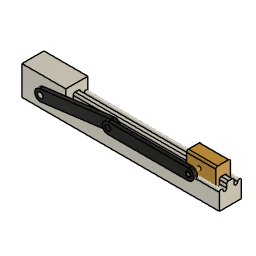
Simple Joint Mechanism_ (Autodesk Fusion 360 design; units mm, degrees)
Autodesk Fusion 360 part; units mm, degrees
sketch "Sketch1" plane through (0, 0, 0) normal (0, 1, 0) x (1, 0, 0) in component "block"
  line L0 (0, 0) -> (120, 0)
  line L1 (120, 0) -> (120, -80)
  line L2 (120, -80) -> (0, -80)
  line L3 (0, -80) -> (0, 0)
  line L4 (120, 0) -> (540, 0)
  line L5 (540, 0) -> (540, -50)
  line L6 (540, -50) -> (120, -50)
  line L7 (120, -50) -> (120, 0)
  dimension "d1" = 120
  dimension "d2" = 80
  dimension "d3" = 420
  dimension "d4" = 50
  constraint horizontal L0
  constraint vertical L1
  constraint horizontal L2
  constraint vertical L3
  constraint coincident L0.start L3.end
  constraint horizontal L4
  constraint vertical L5
  constraint horizontal L6
  constraint vertical L7
  measures "d1" distance of L0.start L0.end
  measures "d2" distance of L0.start L2.end
  measures "d3" distance of L0.end L4.end
  measures "d4" distance of L0.end L6.end
extrude "Extrude1" add sketch "Sketch1" along normal mid plane 60 makes body 1 in component "block"
sketch "Sketch2" plane through (120, 0, 0) normal (1, 0, 0) x (0, 1, 0) in component "block"
  line L0 (-30, 50) -> (30, 50)
  line L1 (30, 50) -> (30, 80)
  line L2 (30, 80) -> (-30, 80)
  line L3 (-30, 80) -> (-30, 50)
  line L4 (-10, 50) -> (10, 50)
  line L5 (10, 50) -> (10, 60)
  line L6 (10, 60) -> (-10, 60)
  line L7 (-10, 60) -> (-10, 50)
  line L8 (-10, 50) -> (-20, 50)
  line L9 (-20, 50) -> (-20, 40)
  line L10 (-20, 40) -> (-10, 40)
  line L11 (-10, 40) -> (-10, 50)
  line L12 (10, 50) -> (20, 50)
  line L13 (20, 50) -> (20, 40)
  line L14 (20, 40) -> (10, 40)
  line L15 (10, 40) -> (10, 50)
  dimension "d7" = 20
  dimension "d8" = 10
  dimension "d9" = 10
  dimension "d10" = 10
  dimension "d11" = 10
  dimension "d12" = 10
  constraint horizontal L4
  constraint vertical L5
  constraint horizontal L6
  constraint vertical L7
  constraint coincident L0 L4.start
  constraint horizontal L8
  constraint vertical L9
  constraint horizontal L10
  constraint vertical L11
  constraint horizontal L12
  constraint vertical L13
  constraint horizontal L14
  constraint vertical L15
  measures "d7" distance of L4.start L4.end
  measures "d8" distance of L4.start L6.end
  measures "d9" distance of L4.start L8.end
  measures "d10" distance of L4.start L10.end
  measures "d11" distance of L4.end L12.end
  measures "d12" distance of L4.end L14.end
extrude "Extrude2" add sketch "Sketch2" along normal blind 420 contours L0 L4 L5 L6 L7 bodies 1 in component "block"
extrude "Extrude3" cut sketch "Sketch2" along normal blind 420 contours L0 L8 L9 L10 L11 | L0 L12 L13 L14 L15 bodies 1 in component "block"
fillet "Fillet1" radius 5 9 edges at (330, -30, 50) (330, -20, 50) (330, -20, 40) (330, -10, 60) (330, 10, 60) (330, 10, 40) (330, 20, 40) (330, 20, 50) (330, 30, 50) on bodies 1 in component "block"
sketch "Sketch3" plane through (0, 30, 0) normal (0, 1, 0) x (-1, 0, 0) in component "block"
  line L0 (-120, 45) -> (-540, 45)
  line L1 (-540, 45) -> (-540, 0)
  line L2 (-540, 0) -> (0, 0)
  line L3 (0, 0) -> (0, 80)
  line L4 (0, 80) -> (-120, 80)
  line L5 (-120, 80) -> (-120, 45)
  circle A0 centre (-60, 40) radius 7.5
  dimension "d19" = 15
  dimension "d20" = 60
  dimension "d21" = 40
  measures "d19" diameter of A0
  measures "d20" horizontal distance of L2.end A0.centre
  measures "d21" vertical distance of L2.end A0.centre
extrude "Extrude4" add sketch "Sketch3" against normal blind 70 contours A0 bodies 1 in component "block"
sketch "Sketch1 (2)" plane through (0, -30, 0) normal (0, -1, 0) x (1, 0, 0) in component "arm1"
  circle A0 centre (60, 40) radius 7.5
  line L0 (540, 45) -> (120, 45)
  line L1 (120, 45) -> (120, 80)
  line L2 (120, 80) -> (0, 80)
  line L3 (0, 80) -> (0, 0)
  line L4 (0, 0) -> (540, 0)
  line L5 (540, 0) -> (540, 45)
  circle A1 centre (60, 40) radius 7.5
  line L6 (38.7868, 40) -> (60, 18.7868)
  line L7 (60, 18.7868) -> (220, 178.7868)
  line L8 (220, 178.7868) -> (198.7868, 200)
  line L9 (198.7868, 200) -> (38.7868, 40)
  circle A2 centre (198.7868, 178.7868) radius 7.5
  dimension "d24" = 15
  dimension "d25" = 15
  dimension "d26" = 30
  dimension "d27" = 160
  dimension "d28" = 15
  dimension "d29" = 15
  dimension "d30" = 15
  constraint perpendicular L6 L7
  constraint parallel L6 L8
  constraint parallel L7 L9
  measures "d24" distance of A0.centre L6
  measures "d25" distance of A0.centre L7
  measures "d26" distance of L6.start L6.end
  measures "d27" vertical distance of L6.start L8.end
  measures "d28" diameter of A2
  measures "d29" distance of L7 A2.centre
  measures "d30" distance of L8 A2.centre
extrude "Extrude1'" add sketch "Sketch1 (2)" along normal blind 10 separate body contours L1 L2 L6 L7 L9 | L1 L2 L7 L8 L9 makes body 2 in component "arm1"
fillet "Fillet1'" radius 15 4 edges at (220, -35, 178.7868) (198.7868, -35, 200) (38.7868, -35, 40) (60, -35, 18.7868) on bodies 2 in component "arm1"
extrude "Extrude2'" add sketch "Sketch1 (2)" along normal blind 20 contours A2 bodies 2 in component "arm1"
sketch "Sketch1 (3)" plane through (540, 0, 0) normal (1, 0, 0) x (0, 1, 0) in component "slide"
  arc A0 (30, 45) -> (20, 45) centre (25, 45) ccw
  arc A1 (10, 45) -> (20, 45) centre (15, 45) ccw
  line L0 (10, 45) -> (10, 55)
  arc A2 (10, 55) -> (5, 60) centre (5, 55) ccw
  line L1 (5, 60) -> (-5, 60)
  arc A3 (-5, 60) -> (-10, 55) centre (-5, 55) ccw
  line L2 (-10, 55) -> (-10, 40)
  line L3 (-10, 40) -> (-15, 40)
  arc A4 (-20, 45) -> (-15, 40) centre (-15, 45) ccw
  arc A5 (-20, 45) -> (-30, 45) centre (-25, 45) ccw
  line L4 (-30, 45) -> (-30, 0)
  line L5 (-30, 0) -> (30, 0)
  line L6 (30, 0) -> (30, 45)
  line L7 (-20, 39.856) -> (20, 39.856)
  line L8 (20, 39.856) -> (20, 89.856)
  line L9 (20, 89.856) -> (-20, 89.856)
  line L10 (-20, 89.856) -> (-20, 39.856)
  dimension "d48" = 40
  dimension "d49" = 50
  constraint horizontal L7
  constraint vertical L8
  constraint horizontal L9
  constraint vertical L10
  measures "d48" distance of L7.start L7.end
  measures "d49" distance of L7.start L9.end
extrude "Extrude1''" add sketch "Sketch1 (3)" against normal blind 80 separate body contours A1 L0 A2 L1 A3 L2 L3 A4 L8 L9 L10 makes body 3 in component "slide"
fillet "Fillet1''" radius 5 2 edges at (500, 20, 89.856) (500, -20, 89.856) on bodies 3 in component "slide"
fillet "Fillet2" radius 5 1 edges at (330, -10, 40) on bodies 1 in component "block"
sketch "Sketch2 (2)" plane through (0, -20, 0) normal (0, -1, 0) x (1, 0, 0) in component "slide"
  line L0 (540, 84.856) -> (460, 84.856)
  line L1 (460, 84.856) -> (460, 45)
  line L2 (460, 45) -> (540, 45)
  line L3 (540, 45) -> (540, 84.856)
  circle A0 centre (494.5631, 64.928) radius 5
extrude "Extrude2''" add sketch "Sketch2 (2)" along normal blind 30 contours A0 bodies 3 in component "slide"
sketch "Sketch2 (3)" plane through (0, -30, 0) normal (0, 1, 0) x (-1, 0, 0) in component "arm2"
  circle A0 centre (-60, 40) radius 7.5
  arc A1 (-70.6066, 29.3934) -> (-49.3934, 50.6066) centre (-60, 40) ccw
  line L0 (-49.3934, 50.6066) -> (-188.1802, 189.3934)
  arc A2 (-188.1802, 189.3934) -> (-209.3934, 168.1802) centre (-198.7868, 178.7868) ccw
  line L1 (-209.3934, 168.1802) -> (-70.6066, 29.3934)
  circle A3 centre (-198.7868, 178.7868) radius 7.5
  line L2 (-183.7868, 163.7868) -> (-433.7868, 163.7868)
  line L3 (-433.7868, 163.7868) -> (-433.7868, 193.7868)
  line L4 (-433.7868, 193.7868) -> (-183.7868, 193.7868)
  line L5 (-183.7868, 193.7868) -> (-183.7868, 163.7868)
  dimension "d59" = 250
  dimension "d60" = 30
  dimension "d61" = 15
  dimension "d62" = 15
  constraint horizontal L2
  constraint vertical L3
  constraint horizontal L4
  constraint vertical L5
  measures "d59" distance of L2.start L2.end
  measures "d60" distance of L2.start L4.end
  measures "d61" distance of A2.centre L5
  measures "d62" distance of A2.centre L2
extrude "Extrude2'''" add sketch "Sketch2 (3)" against normal blind 10 separate body contours A2 L1 L2 L3 L4 | L0 A2 L1 L2 L5 | L0 A2 L4 L5 makes body 4 in component "arm2"
fillet "Fillet2'" radius 15 4 edges at (183.7868, -35, 193.7868) (433.7868, -35, 193.7868) (433.7868, -35, 163.7868) (183.7868, -35, 163.7868) on bodies 4 in component "arm2"
hole "Hole2" at (418.7868, -40, 178.7868) direction (0, 1, 0) diameter 15 depth 40 tip angle 118 bodies 4 in component "arm2"
move_body "Move1" bodies 4 to x (1, 0, 0) y (0, 1, 0) z (0, 0, 1) at (0, -10, 0) in component "arm2"
component "arm1" placed x (0.791187, 0, -0.611574) y (0, 1, 0) z (0.611574, 0, 0.791187) at (7.9442, 0, 45.0469)
component "arm2" placed x (1, 0, 0) y (0, 1, 0) z (0, 0, 1) at (75.7763, 0, -113.8588)
component "slide" placed x (1, 0, 0) y (0, 1, 0) z (0, 0, 1) at (0, 0, 0)
component "block" placed x (1, 0, 0) y (0, 1, 0) z (0, 0, 1) at (19.8784, 0, 0)
